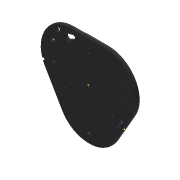
# Autodesk Inventor part: Part4
Saved by Autodesk Inventor 2016 (Build 200138000, 138)
## iProperties
Created: 2016-03-29
Part Number: Part4
Material: ABS Plastic
Document SubType Name: Modeling
Designer: admin
Density: 1 g/cm^3
Appearance: Dark Gray
Author: admin
Autodesk Inventor part; units mm, degrees
ref_plane "YZ Plane" through (0, 0, 0) normal (1, 0, 0) x (0, 1, 0)
ref_plane "XZ Plane" through (0, 0, 0) normal (0, 1, 0) x (-1, 0, 0)
ref_plane "XY Plane" through (0, 0, 0) normal (0, 0, 1) x (1, 0, 0)
sketch "Sketch3" plane through (0, 0, 0) normal (0, 1, 0) x (-1, 0, 0)
  arc A0 (174.3732, -22.7321) -> (67.5, 162.3777) centre (67.5, 38.9711) ccw projected
  line L0 (-67.5, 162.3777) -> (67.5, 162.3777) projected
  arc A1 (-67.5, 162.3777) -> (-174.3732, -22.7321) centre (-67.5, 38.9711) ccw projected
  line L1 (-106.8732, -139.6455) -> (-174.3732, -22.7321) projected
  arc A2 (-106.8732, -139.6455) -> (106.8732, -139.6455) centre (0, -77.9423) ccw projected
  line L2 (174.3732, -22.7321) -> (106.8732, -139.6455) projected
  circle A3 centre (99.5929, -57.5) radius 4.25 projected
  circle A4 centre (0, 115) radius 4.25 projected
  circle A5 centre (-99.5929, -57.5) radius 4.25 projected
  circle A6 centre (-28, -169.4449) radius 2 projected
  circle A7 centre (28, -169.4449) radius 2 projected
  circle A8 centre (-132.7436, 108.9711) radius 2 projected
  circle A9 centre (-160.7436, 60.4737) radius 2 projected
  circle A10 centre (132.7436, 108.9711) radius 2 projected
  circle A11 centre (160.7436, 60.4737) radius 2 projected
  circle A12 centre (0, 0) radius 5 projected
extrude "Extrusion2" add sketch "Sketch3" along normal blind 10
sketch "Sketch4" plane through (0, 10, 0) normal (0, 1, 0) x (1, 0, 0)
  line L0 (-8.5, 160.7449) -> (-8.5, 166.1449) projected
  arc A0 (-7, 167.6449) -> (-8.5, 166.1449) centre (-7, 166.1449) ccw projected
  line L1 (-7, 167.6449) -> (-6, 167.6449) projected
  arc A1 (-8.5, 160.7449) -> (-7, 159.2449) centre (-7, 160.7449) ccw projected
  line L2 (-2, 159.2449) -> (-7, 159.2449) projected
  line L3 (7, 159.2449) -> (2, 159.2449) projected
  arc A2 (7, 159.2449) -> (8.5, 160.7449) centre (7, 160.7449) ccw projected
  line L4 (8.5, 166.1449) -> (8.5, 160.7449) projected
  arc A3 (8.5, 166.1449) -> (7, 167.6449) centre (7, 166.1449) ccw projected
  line L5 (6, 167.6449) -> (7, 167.6449) projected
  line L6 (-6, 167.6449) -> (6, 167.6449)
  line L7 (2, 159.2449) -> (-2, 159.2449)
  constraints: 4 end point, 1 collinear, 1 parallel
extrude "Extrusion3" cut sketch "Sketch4" against normal blind 10
pattern_circular "Circular Pattern1" count 3 over 360 about axis through (0, 0, 0) along (0, 1, 0) of "Extrusion3"
sketch "Sketch7" plane through (0, 10, 0) normal (0, 1, 0) x (1, 0, 0)
  line L0 (174.3732, 22.7321) -> (106.8732, 139.6455) projected
  line L1 (118.645, 82.3561) -> (130.645, 61.5715) construction
  line L2 (117.1295, 81.4811) -> (129.1295, 60.6965)
  line L3 (132.1606, 62.4465) -> (120.1606, 83.2311)
  arc A0 (120.1606, 83.2311) -> (117.1295, 81.4811) centre (118.645, 82.3561) ccw
  arc A1 (129.1295, 60.6965) -> (132.1606, 62.4465) centre (130.645, 61.5715) ccw
  line L4 (140.6232, 81.1888) -> (142.3209, 82.169)
  point P0 (124.645, 71.9638)
  dimension "d89" = 3.5
  dimension "d90" = 16.7
  dimension "d91" = 12
  dimension "d92" = 12
  constraints: 10 end point, 4 point on circle, 4 tangent, 2 centre point, 2 midpoint, 2 parallel, 1 perpendicular
  measures "d89" diameter of A1
  measures "d90" distance between parallel lines of L0 L3
  measures "d91" distance from line of L1.end L4
  measures "d92" distance from line of L1.start L4
extrude "Extrusion5" cut sketch "Sketch7" against normal blind 10
sketch "Sketch8" plane through (0, 0, 0) normal (0, -1, 0) x (1, 0, 0)
  line L0 (-143.4591, 73.0112) -> (-148.1357, 75.7112) projected
  line L1 (111.7912, -85.3273) -> (117.507, -88.6273)
  line L2 (117.507, -88.6273) -> (135.507, -57.4504)
  line L3 (135.507, -57.4504) -> (129.7912, -54.1504)
  line L4 (129.7912, -54.1504) -> (111.7912, -85.3273)
  line L5 (113.117, -85.5154) -> (114.6756, -86.4152) projected
  line L6 (130.617, -55.2045) -> (132.1756, -56.1043) projected
  line L7 (159.7101, -2.7194) -> (82.2101, -136.9533) projected
  line L8 (132.7855, -60.2093) -> (118.5355, -84.891) projected
  circle A0 centre (114.6491, -86.9773) radius 3.3
  circle A1 centre (132.6491, -55.8004) radius 3.3
  line L9 (132.1606, -62.4465) -> (120.1606, -83.2311) projected
  dimension "d155" = 6.6
  dimension "d25" = 0.5
  dimension "d26" = 0.5
  dimension "d156" = 0.4
  constraints: 8 end point, 3 parallel, 2 midpoint, 1 perpendicular, 6 other
  measures "d25" distance between parallel lines of L3 L6
  measures "d26" distance between parallel lines of L5 L1
  measures "d156" distance between parallel lines of L9 L2
extrude "Extrusion6" cut sketch "Sketch8" against normal blind 6.3
sketch "Sketch11" plane through (0, 10, 0) normal (0, 1, 0) x (1, 0, 0)
  circle A0 centre (99.5929, 57.5) radius 4.25 projected
extrude "Extrusion9" add sketch "Sketch11" against normal up to surface (10 mm away)
pattern_circular "Circular Pattern2" count 3 over 360 about axis through (0, 0, 0) along (0, 1, 0) of "Extrusion9"
sketch "Sketch12" plane through (0, 0, 0) normal (0, -1, 0) x (1, 0, 0)
  arc A0 (-106.8732, -139.6455) -> (106.8732, -139.6455) centre (0, -77.9423) ccw projected
  arc A1 (-23, 159.1777) -> (-19.8, 162.3777) centre (-23, 162.3777) ccw projected
  line L0 (67.5, 162.3777) -> (-19.8, 162.3777) projected
  arc A2 (174.3732, -22.7321) -> (67.5, 162.3777) centre (67.5, 38.9711) ccw projected
  line L1 (106.8732, -139.6455) -> (174.3732, -22.7321) projected
  arc A3 (-106.8732, -139.6455) -> (106.8732, -139.6455) centre (0, -77.9423) ccw projected
  line L2 (-150.5232, -64.0415) -> (-106.8732, -139.6455) projected
  arc A4 (-150.5232, -64.0415) -> (-149.3519, -59.6702) centre (-152.1232, -61.2702) ccw projected
  line L3 (-104.1019, -138.0455) -> (-149.3519, -59.6702) projected
  arc A5 (-104.1019, -138.0455) -> (104.1019, -138.0455) centre (0, -77.9423) ccw projected
  line L4 (171.6019, -21.1321) -> (104.1019, -138.0455) projected
  arc A6 (171.6019, -21.1321) -> (67.5, 159.1777) centre (67.5, 38.9711) ccw projected
  line L5 (-23, 159.1777) -> (67.5, 159.1777) projected
  arc A7 (-150.8241, -63.5202) -> (-150.8241, -60.5202) centre (-153.4222, -62.0202) ccw projected
  line L6 (-150.8241, -60.5202) -> (-173.0741, -21.9821) projected
  arc A8 (-67.5, 160.8777) -> (-173.0741, -21.9821) centre (-67.5, 38.9711) ccw projected
  line L7 (-67.5, 160.8777) -> (-23, 160.8777) projected
  arc A9 (-23, 160.8777) -> (-20.4019, 162.3777) centre (-23, 163.8777) ccw projected
  line L8 (-19.8, 162.3777) -> (-20.4019, 162.3777) projected
  arc A10 (-23, 159.1777) -> (-19.8, 162.3777) centre (-23, 162.3777) ccw projected
  line L9 (-67.5, 159.1777) -> (-23, 159.1777) projected
  arc A11 (-67.5, 159.1777) -> (-171.6019, -21.1321) centre (-67.5, 38.9711) ccw projected
  line L10 (-149.3519, -59.6702) -> (-171.6019, -21.1321) projected
  arc A12 (-150.5232, -64.0415) -> (-149.3519, -59.6702) centre (-152.1232, -61.2702) ccw projected
  line L11 (-150.8241, -63.5202) -> (-150.5232, -64.0415) projected
extrude "Extrusion10" cut sketch "Sketch12" against normal blind 3 contours L2 A4 L3 A5 L4 A6 L5 A1 L0 A2 L1 A0 | L11 A7 L6 A8 L7 A9 L8 A1 L9 A11 L10 A4
sketch "Sketch13" plane through (0, 0, 0) normal (0, -1, 0) x (1, 0, 0)
  arc A0 (-23, 160.8777) -> (-20.4019, 162.3777) centre (-23, 163.8777) ccw projected
  line L0 (-67.5, 162.3777) -> (-20.4019, 162.3777) projected
  arc A1 (-67.5, 162.3777) -> (-174.3732, -22.7321) centre (-67.5, 38.9711) ccw projected
  line L1 (-150.8241, -63.5202) -> (-174.3732, -22.7321) projected
  arc A2 (-150.8241, -63.5202) -> (-150.8241, -60.5202) centre (-153.4222, -62.0202) ccw projected
  line L2 (-150.8241, -60.5202) -> (-173.0741, -21.9821) projected
  arc A3 (-67.5, 160.8777) -> (-173.0741, -21.9821) centre (-67.5, 38.9711) ccw projected
  line L3 (-67.5, 160.8777) -> (-23, 160.8777) projected
  point P0 (0, 0)
extrude "Extrusion11" cut sketch "Sketch13" against normal blind 10
sketch "Sketch14" plane through (0, 0, 0) normal (0, -1, 0) x (1, 0, 0)
  line L0 (67.5, 159.1777) -> (-67.5, 159.1777) projected
  line L1 (-171.6019, -21.1321) -> (-104.1019, -138.0455) projected
  circle A0 centre (-61.5, 153.3777) radius 1.65
  circle A1 centre (-29, 153.3777) radius 1.65
  circle A2 centre (-163.5789, -23.4283) radius 1.65
  circle A3 centre (-147.3289, -51.5741) radius 1.65
  line L2 (-171.6019, -21.1321) -> (-171, -20.7846)
  dimension "d47" = 3.3
  dimension "d48" = 3.3
  dimension "d49" = 3.3
  dimension "d50" = 3.3
  dimension "d51" = 5.8
  dimension "d52" = 5.8
  dimension "d53" = 5.8
  dimension "d54" = 5.8
  dimension "d55" = 6
  dimension "d56" = 32.5
  dimension "d57" = 6
  dimension "d58" = 32.5
  constraints: 4 centre point, 2 end point, 1 perpendicular
  measures "d47" diameter of A0
  measures "d48" diameter of A1
  measures "d49" diameter of A2
  measures "d50" diameter of A3
  measures "d51" distance from line of L0 A0.centre
  measures "d52" distance from line of L0 A1.centre
  measures "d53" distance from line of L1 A2.centre
  measures "d54" distance from line of L1 A3.centre
  measures "d55" distance from line of A2.centre L2
  measures "d56" distance of A3.centre A2.centre
  measures "d57" horizontal distance of A0.centre L0.end
  measures "d58" distance of A1.centre A0.centre
extrude "Extrusion12" cut sketch "Sketch14" against normal blind 10
thread "Thread1" size "M3.5x0.6" class "6H" standard "ANSI Metric M Profile" full length
thread "Thread2" size "M3.5x0.6" class "6H" standard "ANSI Metric M Profile" full length
thread "Thread3" size "M3.5x0.6" class "6H" standard "ANSI Metric M Profile" full length
thread "Thread4" size "M3.5x0.6" class "6H" standard "ANSI Metric M Profile" full length
sketch "Sketch15" plane through (0, 0, 0) normal (0, -1, 0) x (1, 0, 0)
  circle A0 centre (-141.4725, -29.7177) radius 1.5 projected
  circle A1 centre (-96.4725, -107.66) radius 1.5 projected
  circle A2 centre (20.4409, -40.16) radius 1.5 projected
  circle A3 centre (-24.5591, 37.7823) radius 1.5 projected
  circle A4 centre (-141.4725, -29.7177) radius 1.5
  circle A5 centre (-96.4725, -107.66) radius 1.5
  circle A6 centre (20.4409, -40.16) radius 1.5
  circle A7 centre (-24.5591, 37.7823) radius 1.5
  dimension "d69" = 3
  dimension "d70" = 3
  dimension "d71" = 3
  dimension "d72" = 3
  constraints: 4 centre point, 4 coincident
  measures "d69" diameter of A4
  measures "d70" diameter of A5
  measures "d71" diameter of A6
  measures "d72" diameter of A7
sketch "Sketch16" plane through (0, 10, 0) normal (0, 1, 0) x (1, 0, 0)
  line L0 (-84.0891, -131.0548) -> (-64.906, -136.1301) projected
  line L1 (-59.5815, -122.9515) -> (-76.9063, -113.2766) projected
  arc A0 (-64.906, -136.1301) -> (-59.5815, -122.9515) centre (-63.0739, -129.2054) ccw projected
  arc A1 (-76.9063, -113.2766) -> (-84.0891, -131.0548) centre (-81.6176, -121.7132) ccw projected
extrude "Extrusion14" cut sketch "Sketch16" against normal blind 10
sketch "Sketch17" plane through (0, 0, 0) normal (0, -1, 0) x (1, 0, 0)
  arc A0 (-59.5815, 122.9515) -> (-64.906, 136.1301) centre (-63.0739, 129.2054) ccw projected
  line L0 (-59.5815, 122.9515) -> (-76.9063, 113.2766) projected
  arc A1 (-84.0891, 131.0548) -> (-76.9063, 113.2766) centre (-81.6176, 121.7132) ccw projected
  line L1 (-84.0891, 131.0548) -> (-64.906, 136.1301) projected
  arc A2 (-57.1437, 118.5861) -> (-66.1849, 140.9638) centre (-63.0739, 129.2054) ccw
  line L2 (-57.1437, 118.5861) -> (-74.4684, 108.9112)
  arc A3 (-85.368, 135.8885) -> (-74.4684, 108.9112) centre (-81.6176, 121.7132) ccw
  line L3 (-85.368, 135.8885) -> (-66.1849, 140.9638)
  dimension "d85" = 5
  constraints: 4 end point, 4 point on circle, 2 centre point, 3 other
  measures "d85" distance between parallel lines of L1 L3
extrude "Extrusion15" cut sketch "Sketch17" against normal blind 3.1
sketch "Sketch20" plane through (0, 0, 0) normal (0, -1, 0) x (1, 0, 0)
  circle A0 centre (131.6623, -15.3935) radius 1.5
  circle A1 centre (116.6623, -41.3742) radius 1.5
  circle A2 centre (94.1623, -80.3454) radius 1.5
  circle A3 centre (79.1623, -106.3262) radius 1.5
  circle A4 centre (-150, 86.6025) radius 16.9314
  circle A5 centre (150, 86.6025) radius 16.9314
  circle A6 centre (0, -173.2051) radius 16.9314
  arc A7 (-95.0309, -137.8544) -> (97.2895, -134.1124) centre (0, -77.9423) ccw
  line L0 (164.7895, -17.199) -> (97.2895, -134.1124)
  arc A8 (164.7895, -17.199) -> (148.0526, 117.2757) centre (67.5, 38.9711) ccw
  spline S0 degree 3 poles (115.8849, 129.2462) (118.7543, 129.4972) (121.6508, 129.4369) (129.4075, 128.4318) (134.1872, 126.8785) (142.0389, 122.5943) (145.2626, 120.1458) (148.0526, 117.2757) knots 0 0 0 0 0.864085 0.864085 2.346474 2.346474 3.547291 3.547291 3.547291 3.547291
  line L1 (16.2499, 120.5292) -> (115.8849, 129.2462)
  arc A9 (16.2499, 120.5292) -> (-65.1861, 94.0714) centre (32.8394, -69.0896) ccw
  arc A10 (-113.6521, 118.9106) -> (-65.1861, 94.0714) centre (-81.6176, 121.7132) ccw
  line L2 (-114.1919, 125.08) -> (-113.6521, 118.9106)
  spline S1 degree 3 poles (-129.6881, 132.5285) (-128.6392, 133.2256) (-127.4577, 133.7226) (-124.6132, 134.3272) (-122.9156, 134.2633) (-119.9531, 133.3948) (-118.662, 132.6875) (-116.4082, 130.7216) (-115.4815, 129.4246) (-114.517, 127.0608) (-114.2791, 126.077) (-114.1919, 125.08) knots 0 0 0 0 0.377832 0.377832 0.872407 0.872407 1.30398 1.30398 1.769607 1.769607 2.069845 2.069845 2.069845 2.069845
  arc A11 (-129.6881, 132.5285) -> (-164.7895, -17.199) centre (-67.5, 38.9711) ccw
  line L3 (-152.5179, -38.4539) -> (-164.7895, -17.199)
  ellipse E0 centre (-149.9204, -36.9521) end of major axis (-149.7401, -39.949) minor radius 3 (-152.5179, -38.4539) -> (-149.5846, -39.9356) ccw
  spline S2 degree 3 poles (-127.1077, -51.2846) (-128.2027, -49.388) (-129.5704, -47.6488) (-133.191, -44.1975) (-135.5857, -42.6356) (-140.3864, -40.6376) (-142.7348, -40.0667) (-146.6022, -39.7464) (-148.1016, -39.7685) (-149.5846, -39.9356) knots -2.664619 -2.664619 -2.664619 -2.664619 -2.007618 -2.007618 -1.16409 -1.16409 -0.447727 -0.447727 0 0 0 0
  line L4 (-93.5522, -109.4044) -> (-127.1077, -51.2846)
  ellipse E1 centre (-113.4969, -120.8871) end of major axis (-91.2536, -126.8472) minor radius 23 (-94.914, -134.4811) -> (-93.5522, -109.4044) ccw
  spline S3 degree 3 poles (-95.0309, -137.8544) (-95.2526, -137.5027) (-95.4002, -137.1045) (-95.5315, -136.219) (-95.486, -135.7279) (-95.2317, -134.9913) (-95.0911, -134.7228) (-94.914, -134.4811) knots 0 0 0 0 0.347927 0.347927 0.749203 0.749203 1 1 1 1
  circle A12 centre (100, 115.4701) radius 9.6924
  circle A13 centre (50, -144.3376) radius 9.6924
  circle A14 centre (150, 28.8675) radius 9.6924
  circle A15 centre (-150, 28.8675) radius 9.6924
  circle A16 centre (-50, -144.3376) radius 9.6924
  constraints: 2 other
hole "Hole1" at (131.6623, 0, -15.3935) at (116.6623, 0, -41.3742) at (94.1623, 0, -80.3454) at (79.1623, 0, -106.3262) direction (0, 1, 0) diameter 2.459 depth 8.5 tip angle 118 thread size "M3x0.5" class "6H" standard "ISO Metric profile"
sketch "Sketch22" plane through (0, 0, 0) normal (0, -1, 0) x (1, 0, 0)
  arc A0 (-67.5, 159.1777) -> (-171.6019, -21.1321) centre (-67.5, 38.9711) ccw projected
  arc A1 (-67.5, 159.1777) -> (-171.6019, -21.1321) centre (-67.5, 38.9711) ccw projected
  circle A2 centre (-137.5, 13.9711) radius 6
  circle A3 centre (-120.5, 127.9711) radius 9
  point P0 (-169.1892, 103.072)
  point P1 (-173.8575, 94.9862)
  dimension "d118" = 18
  dimension "d119" = 89
  dimension "d120" = 53
  dimension "d121" = 12
  dimension "d122" = 25
  dimension "d123" = 70
  constraints: 2 centre point
  measures "d118" diameter of A3
  measures "d119" vertical distance of A1.centre A3.centre
  measures "d120" horizontal distance of A0.centre A3.centre
  measures "d121" diameter of A2
  measures "d122" vertical distance of A0.centre A2.centre
  measures "d123" horizontal distance of A0.centre A2.centre
extrude "Extrusion19" cut sketch "Sketch22" against normal blind 10
sketch "Sketch23" plane through (0, 3, 0) normal (0, -1, 0) x (1, 0, 0)
  arc A0 (-67.5, 160.8777) -> (-173.0741, -21.9821) centre (-67.5, 38.9711) ccw projected
  circle A1 centre (-182.3217, -1.9821) radius 5
  point P0 (0, 0)
  dimension "d126" = 10
  dimension "d127" = 20
  constraints: 1 centre point, 1 point on circle
  measures "d126" diameter of A1
  measures "d127" vertical distance of A0.end A1.centre
extrude "Extrusion20" cut sketch "Sketch23" along normal mid plane 20
sketch "Sketch24" plane through (0, 0, 0) normal (0, -1, 0) x (1, 0, 0)
  circle A0 centre (0, 0) radius 5 projected
  line L0 (111.7912, -85.3273) -> (129.7912, -54.1504) projected
  line L1 (0, 0) -> (120.7912, -69.7388)
  circle A1 centre (95.2628, -55) radius 4.25
  circle A2 centre (0, 110) radius 4.25
  circle A3 centre (-95.2628, -55) radius 4.25
  dimension "d130" = 8.5
  dimension "d131" = 110
  dimension "d134" = 360
  constraints: 3 centre point, 2 end point, 1 midpoint, 1 point on line, 7 other
  measures "d130" diameter of A1
  measures "d131" distance of L1.start A1.centre
extrude "Extrusion21" cut sketch "Sketch24" against normal blind 10 contours A1 L1 | L1 A1 | A2 | A3
sketch "Sketch25" plane through (0, 0, 0) normal (0, -1, 0) x (1, 0, 0)
  point P0 (-150, 28.8675)
  point P1 (-50, -144.3376)
  point P2 (50, -144.3376)
  point P3 (150, 28.8675)
  point P4 (100, 115.4701)
hole "Hole2" at (-150, 0, 28.8675) at (-50, 0, -144.3376) at (50, 0, -144.3376) at (150, 0, 28.8675) at (100, 0, 115.4701) direction (0, 1, 0) diameter 3.242 depth 8.5 tip angle 118 thread size "M4x0.7" class "6H" standard "ANSI Metric M Profile"
sketch "Sketch26" plane through (0, 10, 0) normal (0, 1, 0) x (1, 0, 0)
  arc A0 (-183.9045, -2.7608) -> (-180.5458, 6.6561) centre (-182.3217, 1.9821) ccw projected
  line L0 (-182.3217, 1.9821) -> (-177.6123, 0.3024)
  line L1 (-177.6123, 0.3024) -> (-158.7436, -6.4275)
  circle A1 centre (-177.1414, 0.1344) radius 4.5
  circle A2 centre (-182.3217, 1.9821) radius 5.5
  line L2 (-177.8573, -4.3082) -> (-183.1967, -3.4478)
  line L3 (-174.8842, 4.0274) -> (-179.563, 6.7402)
  dimension "d157" = 9
  dimension "d158" = 11
  constraints: 8 end point, 6 point on circle, 4 tangent, 2 centre point, 1 coincident, 1 collinear, 1 point on line
  measures "d157" diameter of A1
  measures "d158" diameter of A2
extrude "Extrusion22" cut sketch "Sketch26" against normal blind 10
hole "Hole3" at (-141.4725, 0, -29.7177) at (-96.4725, 0, -107.66) at (-24.5591, 0, 37.7823) at (20.4409, 0, -40.16) direction (0, 1, 0) diameter 2.459 depth 8 tip angle 118 thread size "M3x0.5" class "6H" standard "ISO Metric profile"
sketch "Sketch27" plane through (0, 10, 0) normal (0, 1, 0) x (1, 0, 0)
  circle A0 centre (0, 0) radius 5 projected
extrude "Extrusion23" add sketch "Sketch27" against normal blind 10
sketch "Sketch28" plane through (106.8732, 3, -139.6455) normal (0.8660254, 0, -0.5) x (-0.5, 0, -0.8660254)
  point P0 (-67.5, -3)
body "Solid2"
